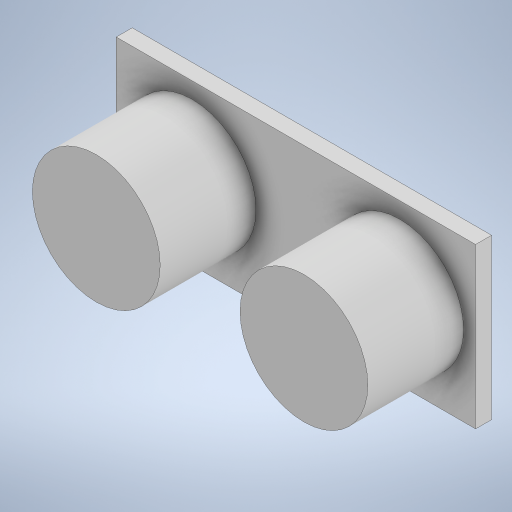
# Autodesk Inventor part: distance
Saved by Autodesk Inventor 2024 (Build 280153000, 153)
## iProperties
Created: 2024-03-14
Part Number: distance
Material: Générique
Document SubType Name: Modeling
Designer: phaly
Density: 1 g/cm^3
Appearance: Par défaut
Author: phaly
Autodesk Inventor part; units mm, degrees
ref_plane "YZ Plane" through (0, 0, 0) normal (1, 0, 0) x (0, 1, 0)
ref_plane "XZ Plane" through (0, 0, 0) normal (0, 1, 0) x (-1, 0, 0)
ref_plane "XY Plane" through (0, 0, 0) normal (0, 0, 1) x (1, 0, 0)
sketch "Esquisse1" plane through (0, 0, 0) normal (0, 0, 1) x (1, 0, 0)
  line L0 (0, 20) -> (45, 20)
  line L1 (45, 20) -> (45, 0)
  line L2 (45, 0) -> (0, 0)
  line L3 (0, 0) -> (0, 20)
  line L4 (-9, 0) -> (54, 0) projected
  line L5 (0, -4) -> (0, 24) projected
  point P0 (0, 0)
  dimension "d0" = 20
  dimension "d1" = 45
  constraints: 8 end point, 2 collinear, 2 parallel, 1 horizontal, 1 perpendicular
  measures "d0" distance of L0.end L1.end
  measures "d1" distance of L0.start L0.end
extrude "Extrusion1" add sketch "Esquisse1" along normal blind 2
sketch "Esquisse2" plane through (0, 0, 2) normal (0, 0, 1) x (1, 0, 0)
  circle A0 centre (9.5, 10) radius 8
  circle A1 centre (35.5, 10) radius 8
  line L0 (0, 10) -> (43.5, 10)
  line L1 (45, 20) -> (0, 20) projected
  line L2 (0, 20) -> (0, 0) projected
  dimension "d6" = 16
  dimension "d4" = 10
  dimension "d5" = 16
  dimension "d7" = 26
  dimension "d8" = 9.5
  constraints: 2 end point, 2 point on line, 1 centre point, 1 horizontal, 1 horizontal alignment, 1 midpoint, 2 other
  measures "d4" distance between parallel lines of L1 L0
  measures "d5" diameter of A0
  measures "d7" distance of point (35.5, 10) A0.centre
  measures "d8" distance from line of L2 A0.centre
extrude "Extrusion2" add sketch "Esquisse2" along normal blind 12
equation "\"d6\" = d5"
